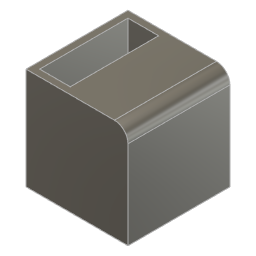
hollowbox v1 (Autodesk Fusion 360 design; units mm, degrees)
Autodesk Fusion 360 part; units mm, degrees
sketch "Sketch1" plane through (0, 0, 0) normal (0, 1, 0) x (1, 0, 0)
  line L0 (0, 0) -> (30, 0)
  line L1 (30, 0) -> (30, -30)
  line L2 (30, -30) -> (0, -30)
  line L3 (0, -30) -> (0, 0)
  dimension "d1" = 30
  dimension "d2" = 30
  constraint horizontal L0
  constraint vertical L1
  constraint horizontal L2
  constraint vertical L3
  constraint coincident L0.start L3.end
  measures "d1" distance of L0.start L0.end
  measures "d2" distance of L0.start L2.end
extrude "Extrude1" add sketch "Sketch1" along normal blind 30
shell "Shell1" thickness 2 removed faces 1 at (10, 30, 10)
sketch "Sketch2" plane through (28, 0, 0) normal (-1, 0, 0) x (0, 0, 1)
  line L0 (2, 2) -> (28, 2)
  line L1 (28, 2) -> (28, 30)
  line L2 (28, 30) -> (2, 30)
  line L3 (2, 30) -> (2, 2)
  line L4 (2, 30) -> (28, 30)
  line L5 (28, 30) -> (28, 26)
  line L6 (28, 26) -> (2, 26)
  line L7 (2, 26) -> (2, 30)
  dimension "d6" = 26
  dimension "d7" = 4
  constraint horizontal L4
  constraint vertical L5
  constraint horizontal L6
  constraint vertical L7
  constraint coincident L2.end L3.start
  measures "d6" distance of L2.end L1.end
  measures "d7" distance of L2.end L6.end
extrude "Extrude2" add sketch "Sketch2" along normal blind 17 contours L1 L2 L3 L4 L5 L6 L7
fillet "Fillet1" radius 4 1 edges at (30, 30, 15)
